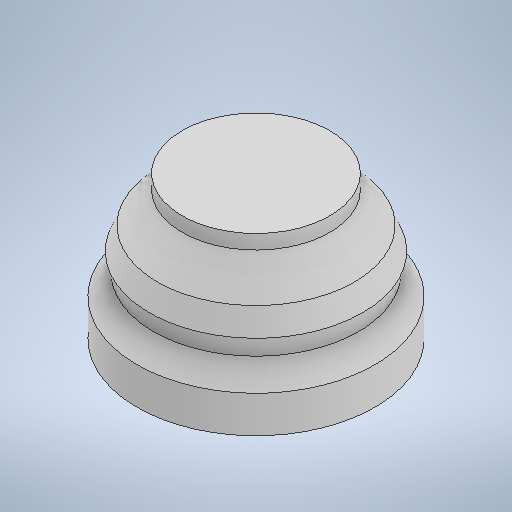
# Autodesk Inventor part: KINGHT BASE 1.0
Saved by Autodesk Inventor 2025.1 (Build 291241000, 241)
## iProperties
Created: 2024-10-24
Part Number: KINGHT BASE 1.0
Material: Genérico
Document SubType Name: Modeling
Designer: Octavio
Density: 1 g/cm^3
Appearance: Valor por defecto
Author: Octavio
Autodesk Inventor part; units mm, degrees
ref_plane "YZ Plane" through (0, 0, 0) normal (1, 0, 0) x (0, 1, 0)
ref_plane "XZ Plane" through (0, 0, 0) normal (0, 1, 0) x (-1, 0, 0)
ref_plane "XY Plane" through (0, 0, 0) normal (0, 0, 1) x (1, 0, 0)
sketch "Boceto2" plane through (0, 0, 0) normal (0, 0, 1) x (1, 0, 0)
  line L0 (-69.9574, 123.8748) -> (72.8997, 123.8748) construction
  line L1 (72.8997, 123.8748) -> (72.8997, -16.6014) construction
  line L2 (72.8997, -16.6014) -> (-69.9574, -16.6014) construction
  line L3 (-69.9574, -16.6014) -> (-69.9574, 123.8748) construction
  line L4 (0, 0) -> (0, 35)
  line L5 (0, 35) -> (0, 0)
  line L6 (-29.0269, 1) -> (-29.0269, 9)
  line L7 (-29.0269, 9) -> (-25.0269, 14)
  line L8 (-25.0269, 14) -> (-26.0269, 18.5)
  line L9 (-26.0269, 18.5) -> (-24.0269, 24)
  line L10 (-24.0269, 24) -> (-21.6269, 27)
  line L11 (-21.6269, 27) -> (-20.0269, 29)
  line L12 (-20.0269, 29) -> (-18.0269, 31.5)
  line L13 (-18.0269, 31.5) -> (-18.0269, 35)
  line L14 (-18.0269, 35) -> (-15.2269, 35)
  line L15 (0, 35) -> (-15.2269, 35)
  line L16 (-18.0269, 35) -> (-15.2269, 35)
  line L17 (0, 0) -> (-29.0269, 0)
  line L18 (-29.0269, 0) -> (-29.0269, 1)
  constraints: 30 end point, 3 point on line, 2 collinear, 2 horizontal, 2 parallel, 2 vertical, 1 perpendicular, 2 other
revolve "Revolución1" add sketch "Boceto2" angle 360 about axis through (0, 0, 0) along (0, 1, 0)
